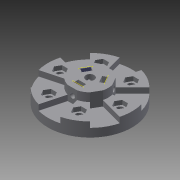
# Autodesk Inventor part: Acoplador MK2
Saved by Autodesk Inventor 2015 (Build 190159000, 159)
## iProperties
Created: 2016-05-12
Part Number: Acoplador MK2
Material: Generic
Document SubType Name: Modeling
Designer: Bruno
Density: 1 g/cm^3
Appearance: Default
Author: Bruno
Autodesk Inventor part; units mm, degrees
ref_plane "YZ Plane" through (0, 0, 0) normal (1, 0, 0) x (0, 1, 0)
ref_plane "XZ Plane" through (0, 0, 0) normal (0, 1, 0) x (-1, 0, 0)
ref_plane "XY Plane" through (0, 0, 0) normal (0, 0, 1) x (1, 0, 0)
sketch "Sketch1" plane through (0, 0, 0) normal (0, 1, 0) x (-1, 0, 0)
  circle A0 centre (0, 0) radius 30
  dimension "d0" = 60
  constraints: 1 centre point, 1 coincident
  measures "d0" diameter of A0
extrude "Extrusion1" add sketch "Sketch1" along normal blind 6
sketch "Sketch2" plane through (0, 6, 0) normal (0, 1, 0) x (1, 0, 0)
  circle A0 centre (0, 0) radius 13
  dimension "d3" = 26
  constraints: 1 centre point, 1 coincident
  measures "d3" diameter of A0
extrude "Extrusion2" add sketch "Sketch2" along normal blind 10
sketch "Sketch4" plane through (0, 6, 0) normal (0, 1, 0) x (1, 0, 0)
  circle A0 centre (0, 0) radius 13 projected
  arc A1 (-12.557, 3.3646) -> (-13, 0) centre (0, 0) ccw
  line L0 (0, 0) -> (-12.557, 3.3646) construction
  line L1 (0, 0) -> (-13, 0) construction
  arc A2 (-9.1924, 9.1924) -> (-12.557, 3.3646) centre (0, 0) ccw
  line L2 (0, 0) -> (-9.1924, 9.1924) construction
  line L3 (0, 0) -> (-12.557, 3.3646) construction
  arc A3 (-3.3646, 12.557) -> (-9.1924, 9.1924) centre (0, 0) ccw
  line L4 (0, 0) -> (-3.3646, 12.557) construction
  line L5 (0, 0) -> (-9.1924, 9.1924) construction
  arc A4 (-21.2132, 21.2132) -> (-28.9778, 7.7646) centre (0, 0) ccw
  line L6 (0, 0) -> (-28.9778, 7.7646) construction
  line L7 (0, 0) -> (30, 0) construction
  line L8 (0, 0) -> (-21.2132, 21.2132) construction
  line L9 (-12.557, 3.3646) -> (-28.9778, 7.7646)
  line L10 (-9.1924, 9.1924) -> (-21.2132, 21.2132)
  arc A5 (-12.557, 3.3646) -> (-12.557, -3.3646) centre (0, 0) ccw
  arc A6 (-28.9778, 7.7646) -> (-28.9778, -7.7646) centre (0, 0) ccw
  line L11 (0, 0) -> (-28.9778, -7.7646) construction
  line L12 (0, 0) -> (-28.9778, 7.7646) construction
  line L13 (-12.557, -3.3646) -> (-28.9778, -7.7646)
  line L14 (-12.557, 3.3646) -> (-28.9778, 7.7646)
  arc A7 (-12.557, -3.3646) -> (-9.1924, -9.1924) centre (0, 0) ccw
  arc A8 (-28.9778, -7.7646) -> (-21.2132, -21.2132) centre (0, 0) ccw
  line L15 (0, 0) -> (-21.2132, -21.2132) construction
  line L16 (0, 0) -> (-28.9778, -7.7646) construction
  line L17 (-9.1924, -9.1924) -> (-21.2132, -21.2132)
  line L18 (-12.557, -3.3646) -> (-28.9778, -7.7646)
  arc A9 (-9.1924, -9.1924) -> (-3.3646, -12.557) centre (0, 0) ccw
  arc A10 (-21.2132, -21.2132) -> (-7.7646, -28.9778) centre (0, 0) ccw
  line L19 (0, 0) -> (-7.7646, -28.9778) construction
  line L20 (0, 0) -> (-21.2132, -21.2132) construction
  line L21 (-3.3646, -12.557) -> (-7.7646, -28.9778)
  line L22 (-9.1924, -9.1924) -> (-21.2132, -21.2132)
  arc A11 (-3.3646, -12.557) -> (3.3646, -12.557) centre (0, 0) ccw
  arc A12 (-7.7646, -28.9778) -> (7.7646, -28.9778) centre (0, 0) ccw
  line L23 (0, 0) -> (7.7646, -28.9778) construction
  line L24 (0, 0) -> (-7.7646, -28.9778) construction
  line L25 (3.3646, -12.557) -> (7.7646, -28.9778)
  line L26 (-3.3646, -12.557) -> (-7.7646, -28.9778)
  arc A13 (3.3646, -12.557) -> (9.1924, -9.1924) centre (0, 0) ccw
  arc A14 (7.7646, -28.9778) -> (21.2132, -21.2132) centre (0, 0) ccw
  line L27 (0, 0) -> (21.2132, -21.2132) construction
  line L28 (0, 0) -> (7.7646, -28.9778) construction
  line L29 (9.1924, -9.1924) -> (21.2132, -21.2132)
  line L30 (3.3646, -12.557) -> (7.7646, -28.9778)
  arc A15 (9.1924, -9.1924) -> (12.557, -3.3646) centre (0, 0) ccw
  arc A16 (21.2132, -21.2132) -> (28.9778, -7.7646) centre (0, 0) ccw
  line L31 (0, 0) -> (28.9778, -7.7646) construction
  line L32 (0, 0) -> (21.2132, -21.2132) construction
  line L33 (12.557, -3.3646) -> (28.9778, -7.7646)
  line L34 (9.1924, -9.1924) -> (21.2132, -21.2132)
  arc A17 (12.557, -3.3646) -> (12.557, 3.3646) centre (0, 0) ccw
  arc A18 (28.9778, -7.7646) -> (28.9778, 7.7646) centre (0, 0) ccw
  line L35 (0, 0) -> (28.9778, 7.7646) construction
  line L36 (0, 0) -> (28.9778, -7.7646) construction
  line L37 (12.557, 3.3646) -> (28.9778, 7.7646)
  line L38 (12.557, -3.3646) -> (28.9778, -7.7646)
  arc A19 (12.557, 3.3646) -> (9.1924, 9.1924) centre (0, 0) ccw
  arc A20 (28.9778, 7.7646) -> (21.2132, 21.2132) centre (0, 0) ccw
  line L39 (0, 0) -> (21.2132, 21.2132) construction
  line L40 (0, 0) -> (28.9778, 7.7646) construction
  line L41 (9.1924, 9.1924) -> (21.2132, 21.2132)
  line L42 (12.557, 3.3646) -> (28.9778, 7.7646)
  arc A21 (9.1924, 9.1924) -> (3.3646, 12.557) centre (0, 0) ccw
  arc A22 (21.2132, 21.2132) -> (7.7646, 28.9778) centre (0, 0) ccw
  line L43 (0, 0) -> (7.7646, 28.9778) construction
  line L44 (0, 0) -> (21.2132, 21.2132) construction
  line L45 (3.3646, 12.557) -> (7.7646, 28.9778)
  line L46 (9.1924, 9.1924) -> (21.2132, 21.2132)
  arc A23 (3.3646, 12.557) -> (-3.3646, 12.557) centre (0, 0) ccw
  arc A24 (7.7646, 28.9778) -> (-7.7646, 28.9778) centre (0, 0) ccw
  line L47 (0, 0) -> (-7.7646, 28.9778) construction
  line L48 (0, 0) -> (7.7646, 28.9778) construction
  line L49 (-3.3646, 12.557) -> (-7.7646, 28.9778)
  line L50 (3.3646, 12.557) -> (7.7646, 28.9778)
  arc A25 (-3.3646, 12.557) -> (-9.1924, 9.1924) centre (0, 0) ccw
  arc A26 (-7.7646, 28.9778) -> (-21.2132, 21.2132) centre (0, 0) ccw
  line L51 (0, 0) -> (-21.2132, 21.2132) construction
  line L52 (0, 0) -> (-7.7646, 28.9778) construction
  line L53 (-9.1924, 9.1924) -> (-21.2132, 21.2132)
  line L54 (-3.3646, 12.557) -> (-7.7646, 28.9778)
  dimension "d12" = 15
  dimension "d13" = 30
  dimension "d14" = 30
  dimension "d15" = 30
  dimension "d16" = 165
  dimension "d17" = 30
  dimension "d20" = 360
  constraints: 110 end point, 52 point on circle, 26 centre point, 4 coincident, 1 collinear, 1 equal length, 1 horizontal, 1 horizontal alignment, 146 other
  measures "d12" angle of L0 L1
  measures "d13" angle of L2 L3
  measures "d14" angle of L4 L5
  measures "d15" radius of A4
  measures "d16" angle of L7 L6
  measures "d17" angle of L8 L6
extrude "Extrusion3" add sketch "Sketch4" along normal blind 4 contours A0 L41 A20 L37 | L33 A16 L29 A0 | A0 L49 A24 L45 | L25 A12 L21 A0 | A0 L9 A4 L10 | L17 A8 L13 A0
sketch "Sketch6" plane through (0, 16, 0) normal (0, 1, 0) x (1, 0, 0)
  line L0 (-12.557, -3.3646) -> (-12.557, 3.3646)
  arc A0 (-12.557, 3.3646) -> (-12.557, -3.3646) centre (0, 0) ccw
  line L1 (-3.3646, -12.557) -> (-9.1924, -9.1924)
  arc A1 (-9.1924, -9.1924) -> (-3.3646, -12.557) centre (0, 0) ccw
  line L2 (9.1924, -9.1924) -> (3.3646, -12.557)
  arc A2 (3.3646, -12.557) -> (9.1924, -9.1924) centre (0, 0) ccw
  line L3 (12.557, 3.3646) -> (12.557, -3.3646)
  arc A3 (12.557, -3.3646) -> (12.557, 3.3646) centre (0, 0) ccw
  line L4 (3.3646, 12.557) -> (9.1924, 9.1924)
  arc A4 (9.1924, 9.1924) -> (3.3646, 12.557) centre (0, 0) ccw
  line L5 (-9.1924, 9.1924) -> (-3.3646, 12.557)
  arc A5 (-3.3646, 12.557) -> (-9.1924, 9.1924) centre (0, 0) ccw
  dimension "d30" = 360
  constraints: 12 end point, 12 point on circle, 6 centre point, 1 coincident, 1 vertical, 31 other
sketch "Sketch7" plane through (0, 10, 0) normal (0, 1, 0) x (1, 0, 0)
  line L0 (0, 0) -> (0, 21.5)
  circle A0 centre (0, 21.5) radius 2.5
  circle A1 centre (-18.6195, 10.75) radius 2.5
  circle A2 centre (-18.6195, -10.75) radius 2.5
  circle A3 centre (0, -21.5) radius 2.5
  circle A4 centre (18.6195, -10.75) radius 2.5
  circle A5 centre (18.6195, 10.75) radius 2.5
  dimension "d32" = 21.5
  dimension "d33" = 5
  dimension "d36" = 360
  constraints: 6 centre point, 2 end point, 1 coincident, 1 vertical, 13 other
  measures "d32" distance of L0.start L0.end
  measures "d33" diameter of A0
extrude "Extrusion4" cut sketch "Sketch7" against normal blind 10
extrude "Extrusion5" cut sketch "Sketch6" against normal blind 10
sketch "Sketch8" plane through (0, 16, 0) normal (0, 1, 0) x (1, 0, 0)
  circle A0 centre (0, 0) radius 3
  dimension "d42" = 6
  constraints: 1 centre point, 1 coincident
  measures "d42" diameter of A0
extrude "Extrusion6" cut sketch "Sketch8" against normal blind 16
sketch "Sketch9" plane through (0, 0, 0) normal (0, -1, 0) x (1, 0, 0)
  circle A0 centre (0, 0) radius 8.7
  dimension "d45" = 17.4
  constraints: 1 centre point, 1 coincident
  measures "d45" diameter of A0
extrude "Extrusion7" cut sketch "Sketch9" against normal blind 3
sketch "Sketch10" plane through (0, 10, 0) normal (0, 1, 0) x (1, 0, 0)
  circle A0 centre (-18.6195, 10.75) radius 2.5 projected
  line L0 (-21.8695, 12.6264) -> (-18.6195, 14.5028)
  line L1 (-18.6195, 14.5028) -> (-15.3695, 12.6264)
  line L2 (-15.3695, 12.6264) -> (-15.3695, 8.8736)
  line L3 (-15.3695, 8.8736) -> (-18.6195, 6.9972)
  line L4 (-18.6195, 6.9972) -> (-21.8695, 8.8736)
  line L5 (-21.8695, 8.8736) -> (-21.8695, 12.6264)
  line L6 (-21.8695, -12.6264) -> (-21.8695, -8.8736)
  line L7 (-21.8695, -8.8736) -> (-18.6195, -6.9972)
  line L8 (-18.6195, -6.9972) -> (-15.3695, -8.8736)
  line L9 (-15.3695, -8.8736) -> (-15.3695, -12.6264)
  line L10 (-15.3695, -12.6264) -> (-18.6195, -14.5028)
  line L11 (-18.6195, -14.5028) -> (-21.8695, -12.6264)
  line L12 (0, -25.2528) -> (-3.25, -23.3764)
  line L13 (-3.25, -23.3764) -> (-3.25, -19.6236)
  line L14 (-3.25, -19.6236) -> (0, -17.7472)
  line L15 (0, -17.7472) -> (3.25, -19.6236)
  line L16 (3.25, -19.6236) -> (3.25, -23.3764)
  line L17 (3.25, -23.3764) -> (0, -25.2528)
  line L18 (21.8695, -12.6264) -> (18.6195, -14.5028)
  line L19 (18.6195, -14.5028) -> (15.3695, -12.6264)
  line L20 (15.3695, -12.6264) -> (15.3695, -8.8736)
  line L21 (15.3695, -8.8736) -> (18.6195, -6.9972)
  line L22 (18.6195, -6.9972) -> (21.8695, -8.8736)
  line L23 (21.8695, -8.8736) -> (21.8695, -12.6264)
  line L24 (21.8695, 12.6264) -> (21.8695, 8.8736)
  line L25 (21.8695, 8.8736) -> (18.6195, 6.9972)
  line L26 (18.6195, 6.9972) -> (15.3695, 8.8736)
  line L27 (15.3695, 8.8736) -> (15.3695, 12.6264)
  line L28 (15.3695, 12.6264) -> (18.6195, 14.5028)
  line L29 (18.6195, 14.5028) -> (21.8695, 12.6264)
  line L30 (0, 25.2528) -> (3.25, 23.3764)
  line L31 (3.25, 23.3764) -> (3.25, 19.6236)
  line L32 (3.25, 19.6236) -> (0, 17.7472)
  line L33 (0, 17.7472) -> (-3.25, 19.6236)
  line L34 (-3.25, 19.6236) -> (-3.25, 23.3764)
  line L35 (-3.25, 23.3764) -> (0, 25.2528)
  circle A1 centre (0, 0) radius 8.7 projected
  line L36 (-15.0195, 8.6715) -> (-18.6195, 6.5931)
  line L37 (-18.6195, 6.5931) -> (-22.2195, 8.6715)
  line L38 (-22.2195, 8.6715) -> (-22.2195, 12.8285)
  line L39 (-22.2195, 12.8285) -> (-18.6195, 14.9069)
  line L40 (-18.6195, 14.9069) -> (-15.0195, 12.8285)
  line L41 (-15.0195, 12.8285) -> (-15.0195, 8.6715)
  line L42 (-15.0195, -8.6715) -> (-15.0195, -12.8285)
  line L43 (-15.0195, -12.8285) -> (-18.6195, -14.9069)
  line L44 (-18.6195, -14.9069) -> (-22.2195, -12.8285)
  line L45 (-22.2195, -12.8285) -> (-22.2195, -8.6715)
  line L46 (-22.2195, -8.6715) -> (-18.6195, -6.5931)
  line L47 (-18.6195, -6.5931) -> (-15.0195, -8.6715)
  line L48 (0, -17.3431) -> (3.6, -19.4215)
  line L49 (3.6, -19.4215) -> (3.6, -23.5785)
  line L50 (3.6, -23.5785) -> (0, -25.6569)
  line L51 (0, -25.6569) -> (-3.6, -23.5785)
  line L52 (-3.6, -23.5785) -> (-3.6, -19.4215)
  line L53 (-3.6, -19.4215) -> (0, -17.3431)
  line L54 (15.0195, -8.6715) -> (18.6195, -6.5931)
  line L55 (18.6195, -6.5931) -> (22.2195, -8.6715)
  line L56 (22.2195, -8.6715) -> (22.2195, -12.8285)
  line L57 (22.2195, -12.8285) -> (18.6195, -14.9069)
  line L58 (18.6195, -14.9069) -> (15.0195, -12.8285)
  line L59 (15.0195, -12.8285) -> (15.0195, -8.6715)
  line L60 (15.0195, 8.6715) -> (15.0195, 12.8285)
  line L61 (15.0195, 12.8285) -> (18.6195, 14.9069)
  line L62 (18.6195, 14.9069) -> (22.2195, 12.8285)
  line L63 (22.2195, 12.8285) -> (22.2195, 8.6715)
  line L64 (22.2195, 8.6715) -> (18.6195, 6.5931)
  line L65 (18.6195, 6.5931) -> (15.0195, 8.6715)
  line L66 (0, 17.3431) -> (-3.6, 19.4215)
  line L67 (-3.6, 19.4215) -> (-3.6, 23.5785)
  line L68 (-3.6, 23.5785) -> (0, 25.6569)
  line L69 (0, 25.6569) -> (3.6, 23.5785)
  line L70 (3.6, 23.5785) -> (3.6, 19.4215)
  line L71 (3.6, 19.4215) -> (0, 17.3431)
  point P0 (-21.8695, 10.75)
  point P1 (-20.2445, -13.5646)
  point P2 (1.625, -24.3146)
  point P3 (21.8695, -10.75)
  point P4 (20.2445, 13.5646)
  point P5 (-1.625, 24.3146)
  point P6 (-15.0195, 10.75)
  point P7 (-16.8195, -7.6323)
  point P8 (-1.8, -18.3823)
  point P9 (15.0195, -10.75)
  point P10 (16.8195, 7.6323)
  point P11 (1.8, 18.3823)
  dimension "d51" = 360
  dimension "d100" = 360
  constraints: 144 end point, 2 midpoint, 1 coincident, 184 other
extrude "Extrusion8" cut sketch "Sketch10" against normal blind 3 contours A0 | L0 L1 L2 L3 L4 L5 | L6 L7 L8 L9 L10 L11 | L12 L13 L14 L15 L16 L17 | L18 L19 L20 L21 L22 L23 | L24 L25 L26 L27 L28 L29 | L30 L31 L32 L33 L34 L35 | L36 L37 L38 L39 L40 L41 | L42 L43 L44 L45 L46 L47 | L48 L49 L50 L51 L52 L53 | L54 L55 L56 L57 L58 L59 | L60 L61 L62 L63 L64 L65 | L66 L67 L68 L69 L70 L71
sketch "Sketch11" plane through (3.3646, 10, 12.557) normal (0.5, 0, 0.8660254) x (0.8660254, 0, -0.5)
  line L0 (0.3646, 6) -> (6.3646, 6) projected
  line L1 (3.3646, 6) -> (3.3646, -4)
  line L2 (6.7293, -4) -> (0, -4) projected
  circle A0 centre (3.3646, 1) radius 1.75
  point P0 (3.3646, -10)
  dimension "d55" = 3.5
  constraints: 3 midpoint, 2 end point, 1 centre point
  measures "d55" diameter of A0
extrude "Extrusion9" cut sketch "Sketch11" against normal blind 13
sketch "Sketch14" plane through (9.1924, 10, -9.1924) normal (0.5, 0, -0.8660254) x (-0.8660254, 0, -0.5)
  line L0 (6.7293, 6) -> (0, 6) projected
  line L1 (3.3646, 6) -> (3.3646, -4)
  line L2 (6.7293, -4) -> (0, -4) projected
  circle A0 centre (3.3646, 1) radius 1.75
  point P0 (3.3646, -10)
  dimension "d64" = 3.5
  constraints: 3 midpoint, 2 end point, 1 centre point
  measures "d64" diameter of A0
extrude "Extrusion12" cut sketch "Sketch14" against normal blind 13
sketch "Sketch16" plane through (-12.557, 16, -3.3646) normal (-1, 0, 0) x (0, 0, 1)
  line L0 (11.1292, -10) -> (-4.3999, -10) projected
  line L1 (3.3646, -10) -> (3.3646, 0)
  line L2 (0.3646, 0) -> (6.3646, 0) projected
  circle A0 centre (3.3646, -5) radius 1.75
  point P0 (3.3646, -16)
  dimension "d67" = 3.5
  constraints: 3 midpoint, 2 end point, 1 centre point
  measures "d67" diameter of A0
extrude "Extrusion13" cut sketch "Sketch16" against normal blind 13
ref_plane "Work Plane1" through (-8.557, 16, -3.3646) normal (-1, 0, 0) x (0, 0, 1)
ref_plane "Work Plane2" through (1.3646, 10, 9.0929) normal (0.5, 0, 0.8660254) x (0.8660254, 0, -0.5)
ref_plane "Work Plane3" through (7.1924, 10, -5.7283) normal (0.5, 0, -0.8660254) x (-0.8660254, 0, -0.5)
sketch "Sketch19" plane through (-8.557, 16, -3.3646) normal (-1, 0, 0) x (0, 0, 1)
  circle A0 centre (3.3646, -5) radius 1.75 projected
  circle A1 centre (3.3646, -5) radius 2.8
  line L0 (3.3646, -5) -> (4.7646, -2.5751)
  line L1 (3.3646, -5) -> (6.1646, -5) construction
  line L2 (6.1646, -3.3834) -> (6.1646, -6.6166)
  line L3 (6.1646, -6.6166) -> (3.3646, -8.2332)
  line L4 (3.3646, -8.2332) -> (0.5646, -6.6166)
  line L5 (0.5646, -6.6166) -> (0.5646, -3.3834)
  line L6 (0.5646, -3.3834) -> (3.3646, -1.7668)
  line L7 (3.3646, -1.7668) -> (6.1646, -3.3834)
  point P0 (3.3646, -16)
  dimension "d77" = 5.6
  dimension "d78" = 60
  constraints: 16 end point, 2 coincident, 1 equal length, 1 horizontal, 1 midpoint, 16 other
  measures "d78" angle of L1 L0
extrude "Extrusion14" cut sketch "Sketch19" against normal blind 3 contours A0 | A1 | L2 L3 A1 | A1 L7 L2 | A1 L6 L7 | L3 L4 A1 | A1 L5 L6 | L4 L5 A1
pattern_circular "Circular Pattern1" count 3 over 360 about axis through (0, -10, 0) along (0, 1, 0) of "Extrusion14"
sketch "Sketch20" plane through (0, 16, 0) normal (0, 1, 0) x (1, 0, 0)
  line L0 (3.3646, -12.557) -> (9.1924, -9.1924) projected
  line L1 (9.1924, 9.1924) -> (3.3646, 12.557) projected
  line L2 (-12.557, 3.3646) -> (-12.557, -3.3646) projected
  line L3 (-8.557, 0) -> (-8.557, -2.8)
  line L4 (-8.557, -2.8) -> (-8.557, 0) projected
  line L5 (-8.557, -2.8) -> (-8.557, 2.8)
  line L6 (-8.557, 2.8) -> (-5.557, 2.8)
  line L7 (-5.557, 2.8) -> (-5.557, -2.8)
  line L8 (-5.557, -2.8) -> (-8.557, -2.8)
  line L9 (-8.557, 0) -> (-8.557, 2.8) projected
  line L10 (6.7034, -6.0106) -> (1.8536, -8.8106)
  line L11 (1.8536, -8.8106) -> (0.3536, -6.2125)
  line L12 (0.3536, -6.2125) -> (5.2034, -3.4125)
  line L13 (5.2034, -3.4125) -> (6.7034, -6.0106)
  line L14 (1.8536, 8.8106) -> (6.7034, 6.0106)
  line L15 (6.7034, 6.0106) -> (5.2034, 3.4125)
  line L16 (5.2034, 3.4125) -> (0.3536, 6.2125)
  line L17 (0.3536, 6.2125) -> (1.8536, 8.8106)
  point P0 (0, 0)
  point P1 (4.2785, 7.4106)
  dimension "d88" = 2.8
  dimension "d89" = 5.6
  dimension "d90" = 3
  dimension "d93" = 360
  constraints: 26 end point, 2 collinear, 2 parallel, 1 perpendicular, 25 other
  measures "d88" distance of L3.start L3.end
  measures "d89" distance of L3.end L5.end
  measures "d90" distance of L5.end L6.end
extrude "Extrusion15" cut sketch "Sketch20" against normal blind 5
body "Solid1"
